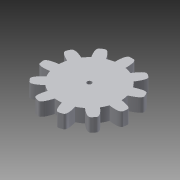
# Autodesk Inventor part: Zahnrad
Saved by Autodesk Inventor 2015 (Build 190159000, 159)
## iProperties
Created: 2015-02-05
Part Number: Zahnrad
Material: ABS-Kunststoff
Document SubType Name: Modeling
Designer: Luki
Density: 1.06 g/cm^3
Appearance: Glatt - weiß
Mass: 4.68821 g
Surface Area: 30.0117 cm^2
Volume: 4.42284 cm^3
Author: Luki
Autodesk Inventor part; units mm, degrees
ref_plane "YZ Plane" through (0, 0, 0) normal (1, 0, 0) x (0, 1, 0)
ref_plane "XZ Plane" through (0, 0, 0) normal (0, 1, 0) x (-1, 0, 0)
ref_plane "XY Plane" through (0, 0, 0) normal (0, 0, 1) x (1, 0, 0)
sketch "Skizze1" plane through (0, 0, 0) normal (0, 0, 1) x (1, 0, 0)
  circle A0 centre (0, 0) radius 14
  dimension "d0" = 28
  constraints: 1 centre point, 1 coincident
  measures "d0" diameter of A0
extrude "Extrusion1" add sketch "Skizze1" along normal blind 6
sketch "Skizze2" plane through (0, 0, 0) normal (0, 0, 1) x (1, 0, 0)
  circle A0 centre (0, 0) radius 14 projected
  line L0 (0, 26.61) -> (0, -26.6017) projected
  line L1 (-26.6, 0) -> (26.6, 0) projected
  circle A1 centre (0, 0) radius 19
  circle A2 centre (0, 0) radius 17
  line L2 (0, 0) -> (5.3529, 18.2304)
  line L3 (0, 0) -> (-5.3529, 18.2304)
  line L4 (0, 0) -> (-2.4352, 18.8433)
  arc A3 (-2.1788, 16.8598) -> (-2.2, 13.8261) centre (7.6946, 15.2739) ccw
  arc A4 (-1.3, 18.9555) -> (-2.1788, 16.8598) centre (1.7974, 16.4245) ccw
  line L5 (-2.3733, 13.7974) -> (0, 13.7974)
  line L6 (0, 13.7974) -> (0, 19)
  line L7 (-1.3, 18.9555) -> (0, 19)
  arc A5 (-2.1788, 16.8598) -> (-2.3733, 13.7974) centre (13.6539, 14.3168) ccw
  arc A6 (-1.3, 18.9555) -> (-2.1788, 16.8598) centre (1.7974, 16.4245) ccw
  line L8 (-2.3733, 13.7974) -> (0, 13.7974)
  line L9 (0, 13.7974) -> (0, 19)
  line L10 (0, 19) -> (-1.3, 18.9555)
  dimension "d4" = 34
  dimension "d3" = 38
  dimension "d5" = 16.364
  dimension "d6" = 16.364
  dimension "d7" = 7.364
  dimension "d8" = 2.2
  dimension "d9" = 1.3
  dimension "d10" = 4
  dimension "d11" = 10
  constraints: 18 end point, 15 point on circle, 5 centre point, 3 point on line, 2 coincident, 2 collinear, 1 concentric, 1 horizontal, 1 perpendicular, 1 tangent, 3 other
  measures "d3" diameter of A1
  measures "d5" angle of L0 L2
  measures "d6" angle of L0 L3
  measures "d7" angle of L0 L4
  measures "d8" distance from line of L0 A0.start
  measures "d9" distance from line of L0 L7.start
  measures "d10" radius of A4
  measures "d11" radius of A3
extrude "Extrusion2" add sketch "Skizze2" along normal blind 6 contours A0 L4 L5 | A3 L4 A0 | A0 A5 A3 | L4 A2 L0 A0 | A0 L0 L5 L4 | A4 L7 L0 A2
mirror "Spiegeln1" about plane through (0, 13.7974, 0) normal (1, 0, 0) of "Extrusion2"
pattern_circular "Runde Anordnung1" count 11 over 360 about axis through (0, 0, -10) along (0, 0, 1) of "Extrusion2", "Spiegeln1"
fillet "Rundung1" radius 1 2 edges at (-1.3, 18.9555, 3) (1.3, 18.9555, 3)
pattern_circular "Runde Anordnung2" count 11 over 360 about axis through (0, 0, -10) along (0, 0, 1) of "Rundung1"
sketch "Skizze3" plane through (0, 0, 0) normal (0, 0, -1) x (-1, 0, 0)
  line L0 (6.5, 6.5) -> (-6.5, 6.5)
  line L1 (-6.5, 6.5) -> (-6.5, -6.5)
  line L2 (-6.5, -6.5) -> (6.5, -6.5)
  line L3 (6.5, -6.5) -> (6.5, 6.5)
  line L4 (6.5, 6.5) -> (-6.5, -6.5) construction
  line L5 (-6.5, 6.5) -> (6.5, -6.5) construction
  point P0 (0, 0)
  dimension "d21" = 13
  dimension "d22" = 13
  constraints: 12 end point, 2 midpoint, 2 parallel, 1 horizontal, 1 perpendicular
  measures "d21" distance between parallel lines of L3 L1
  measures "d22" distance between parallel lines of L0 L2
extrude "Extrusion3" cut sketch "Skizze3" against normal blind 4
sketch "Skizze4" plane through (0, 0, 4) normal (0, 0, -1) x (-1, 0, 0)
  circle A0 centre (0, 0) radius 1
  dimension "d25" = 2
  constraints: 1 centre point, 1 coincident
  measures "d25" diameter of A0
extrude "Extrusion4" cut sketch "Skizze4" against normal blind 3
equation "\"d6\" = d5"
equation "\"d7\" = 0.45 * d6"
equation "\"d22\" = d21"
